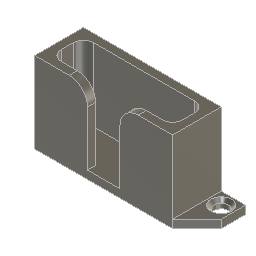
Держатель зажимных клещей (Autodesk Fusion 360 design; units mm, degrees)
Autodesk Fusion 360 part; units mm, degrees
sketch "Sketch1" plane through (0, 0, 0) normal (0, 0, 1) x (1, 0, 0)
  line L0 (4, 2) -> (-4, 2)
  line L1 (-4, 2) -> (-4, -2)
  line L2 (-4, -2) -> (4, -2)
  line L3 (4, -2) -> (4, 2)
  line L4 (4, 2) -> (-4, -2) construction
  line L5 (-4, 2) -> (4, -2) construction
  line L6 (-4, -2) -> (-17, -2)
  line L7 (-17, -2) -> (-17, 10)
  line L8 (-17, 10) -> (0, 10)
  line L9 (-4, 0) -> (-15, 0)
  line L10 (-15, 0) -> (-15, 8)
  line L11 (-15, 8) -> (0, 8)
  line L12 (0, 1.75) -> (0, 22.5)
  line L13 (15, 8) -> (0, 8)
  line L14 (17, 10) -> (0, 10)
  line L15 (17, -2) -> (17, 10)
  line L16 (15, 0) -> (15, 8)
  line L17 (4, 0) -> (15, 0)
  line L18 (4, -2) -> (17, -2)
  line L19 (-17, 10) -> (-23, 10)
  line L20 (-23, 10) -> (-23, 4)
  line L21 (-17, -2) -> (-17, 10)
  circle A0 centre (-20, 7) radius 1.75
  line L22 (-23, 4) -> (-17, -2)
  line L23 (17, 10) -> (23, 10)
  line L24 (23, 10) -> (23, 4)
  line L25 (23, 4) -> (17, -2)
  circle A1 centre (20, 7) radius 1.75
  dimension "d1" = 8
  dimension "d2" = 4
  dimension "d9" = 3.5
  constraint horizontal L0
  constraint perpendicular L0 L1
  constraint parallel L0 L2
  constraint parallel L1 L3
  constraint coincident L4 origin
  constraint coincident L5 origin
  constraint perpendicular L1 L6
  constraint perpendicular L2 L7
  constraint perpendicular L7 L8
  constraint midpoint L1 L9.start
  constraint perpendicular L1 L9
  constraint perpendicular L9 L10
  constraint perpendicular L1 L11
  constraint symmetric L1.end L12 L2.end
  constraint symmetric L6.end L12 L15.start
  constraint symmetric L7.end L12 L14.start
  constraint symmetric L8.end L12 L14.end
  constraint symmetric L9.start L12 L17.start
  constraint symmetric L9.end L12 L16.start
  constraint symmetric L10.end L12 L13.start
  constraint symmetric L11.end L12 L13.end
  constraint horizontal L19
  constraint vertical L20
  constraint vertical L21
  constraint symmetric L12 L19.end L23.end
  constraint symmetric L12 L6.end L15.start
  constraint symmetric L12 A0 A1
  constraint symmetric L12 L20.end L24.end
  measures "d1" distance of L1.end L2.end
  measures "d2" distance of L0.end L1.end
  measures "d9" diameter of A0
extrude "Extrude1" add sketch "Sketch1" along normal blind 2
extrude "Extrude2" add sketch "Sketch1" along normal blind 20 contours L3 L12 L13 L14 L15 L16 L17 L18 | L1 L6 L7 L8 L9 L10 L11 L12 L21
chamfer "Chamfer1" distance 0.8 angle 45 2 edges at (-21.6316, 7.6328, 2) (18.3684, 7.6328, 2)
fillet "Fillet2" radius 4.5 2 edges at (-4, -1, 20) (4, -1, 20)
fillet "Fillet3" radius 2.5 4 edges at (-15, 0, 11) (-15, 8, 11) (15, 8, 11) (15, 0, 11)
